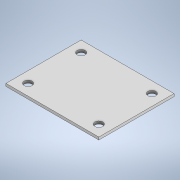
# Autodesk Inventor part: Placa_Rueda_105x85_80x60_3
Saved by Autodesk Inventor 2020 (Build 240168000, 168)
## iProperties
Created: 2022-03-28
Part Number: Placa_Rueda_105x85_80x60_3
Material: Genérico
Document SubType Name: Modeling
Designer: aarco
Density: 1 g/cm^3
Appearance: Valor por defecto
Author: aarco
Autodesk Inventor part; units mm, degrees
ref_plane "YZ Plane" through (0, 0, 0) normal (1, 0, 0) x (0, 1, 0)
ref_plane "XZ Plane" through (0, 0, 0) normal (0, 1, 0) x (-1, 0, 0)
ref_plane "XY Plane" through (0, 0, 0) normal (0, 0, 1) x (1, 0, 0)
sketch "Boceto1" plane through (0, 0, 0) normal (0, 1, 0) x (-1, 0, 0)
  line L0 (52.5, 42.5) -> (-52.5, 42.5)
  line L1 (-52.5, 42.5) -> (-52.5, -42.5)
  line L2 (-52.5, -42.5) -> (52.5, -42.5)
  line L3 (52.5, -42.5) -> (52.5, 42.5)
  line L4 (40, 30) -> (-40, 30)
  line L5 (-40, 30) -> (-40, -30)
  line L6 (-40, -30) -> (40, -30)
  line L7 (40, -30) -> (40, 30)
  line L8 (0, -30) -> (0, -42.5)
  line L9 (52.5, 0) -> (40, 0)
  line L10 (40, 0) -> (0, 0) construction
  line L11 (0, -30) -> (0, 0) construction
  circle A0 centre (40, 30) radius 4.5
  circle A1 centre (40, -30) radius 4.5
  circle A2 centre (-40, -30) radius 4.5
  circle A3 centre (-40, 30) radius 4.5
  dimension "d0" = 105
  dimension "d1" = 85
  dimension "d4" = 80
  dimension "d5" = 60
  dimension "d6" = 9
  dimension "d7" = 9
  dimension "d8" = 9
  dimension "d9" = 9
  constraints: 24 end point, 6 coincident, 4 centre point, 4 midpoint, 4 parallel, 4 perpendicular, 3 horizontal, 1 vertical
  measures "d0" distance of L0.start L0.end
  measures "d1" distance of L2.end L0.start
  measures "d4" distance of L4.start L4.end
  measures "d5" distance of L4.end L5.end
  measures "d6" diameter of A0
  measures "d7" diameter of A1
  measures "d8" diameter of A2
  measures "d9" diameter of A3
extrude "Extrusión1" add sketch "Boceto1" along normal blind 3 contours L3 L9 L7 A0 L4 A3 L5 A2 L6 L8 L2 L1 L0 | L3 L2 L8 L6 A1 L7 L9 | L7 A1 L6 A2 L5 A3 L4 A0
